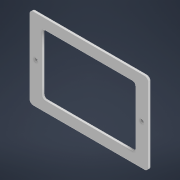
# Autodesk Inventor part: WT-SC01-PLUS_Pannel
Saved by Autodesk Inventor 2021.2 (Build 252289000, 289)
## iProperties
Created: 2024-03-19
Part Number: WT-SC01-PLUS_Pannel
Material: 일반
Document SubType Name: Modeling
Designer: Lee JunHo
Density: 1 g/cm^3
Appearance: 기본값
Author: Lee JunHo
Autodesk Inventor part; units mm, degrees
ref_plane "YZ Plane" through (0, 0, 0) normal (1, 0, 0) x (0, 1, 0)
ref_plane "XZ Plane" through (0, 0, 0) normal (0, 1, 0) x (-1, 0, 0)
ref_plane "XY Plane" through (0, 0, 0) normal (0, 0, 1) x (1, 0, 0)
sketch "스케치1" plane through (0, 0, 0) normal (0, 0, 1) x (1, 0, 0)
  line L0 (44.2668, -29.4131) -> (-41.7332, -29.4131)
  line L1 (-57.1332, -35.7931) -> (-57.1332, 37.0069)
  line L2 (-41.7332, 30.5869) -> (44.2668, 30.5869)
  arc A0 (-53.5332, 40.6069) -> (-57.1332, 37.0069) centre (-53.5332, 37.0069) ccw
  line L3 (-53.5332, -39.3931) -> (56.0668, -39.4131)
  arc A1 (-41.7332, 30.5869) -> (-44.7332, 27.5869) centre (-41.7332, 27.5869) ccw
  arc A2 (56.0668, -39.4131) -> (59.6668, -35.8131) centre (56.0668, -35.8131) ccw
  arc A3 (47.2668, 27.5869) -> (44.2668, 30.5869) centre (44.2668, 27.5869) ccw
  circle A4 centre (-50.9332, 0.5869) radius 1.8
  arc A5 (44.2668, -29.4131) -> (47.2668, -26.4131) centre (44.2668, -26.4131) ccw
  arc A6 (59.6668, 36.9869) -> (56.0668, 40.5869) centre (56.0668, 36.9869) ccw
  circle A7 centre (53.4668, 0.5869) radius 1.8
  line L4 (56.0668, 40.5869) -> (-53.5332, 40.6069)
  arc A8 (-57.1332, -35.7931) -> (-53.5332, -39.3931) centre (-53.5332, -35.7931) ccw
  arc A9 (-44.7332, -26.4131) -> (-41.7332, -29.4131) centre (-41.7332, -26.4131) ccw
  line L5 (47.2668, 27.5869) -> (47.2668, -26.4131)
  line L6 (59.6668, -35.8131) -> (59.6668, 36.9869)
  line L7 (-44.7332, 27.5869) -> (-44.7332, -26.4131)
  point P0 (0, 0)
  constraints: 16 end point, 16 point on circle, 10 centre point
extrude "돌출1" add sketch "스케치1" along normal blind 2
